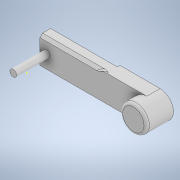
# Autodesk Inventor part: s.Strikrt
Saved by Autodesk Inventor 2020 (Build 240168000, 168)
## iProperties
Created: 2020-04-14
Part Number: s.Strikrt
Material: Generic
Document SubType Name: Modeling
Designer: Darugar
Density: 1 g/cm^3
Appearance: Default
Author: Darugar
Autodesk Inventor part; units mm, degrees
ref_plane "YZ Plane" through (0, 0, 0) normal (1, 0, 0) x (0, 1, 0)
ref_plane "XZ Plane" through (0, 0, 0) normal (0, 1, 0) x (-1, 0, 0)
ref_plane "XY Plane" through (0, 0, 0) normal (0, 0, 1) x (1, 0, 0)
sketch "Sketch1" plane through (0, 0, 0) normal (0, 0, 1) x (1, 0, 0)
  point P0 (0, 0)
sketch "Sketch2" plane through (0, 0, 0) normal (0, 0, 1) x (1, 0, 0)
  line L0 (0, 0) -> (50, 0)
  line L1 (50, 0) -> (50, 20)
  line L2 (50, 20) -> (0, 20)
  line L3 (0, 20) -> (0, 0)
  dimension "d0" = 50
  dimension "d1" = 20
  constraints: 8 end point, 2 parallel, 1 horizontal, 1 perpendicular
  measures "d0" distance of L2.end L1.end
  measures "d1" distance of L1.end L0.end
extrude "Extrusion1" add sketch "Sketch2" along normal blind 10
sketch "Sketch3" plane through (0, 0, 10) normal (0, 0, 1) x (1, 0, 0)
  line L0 (0, 20) -> (0, 0) projected
  line L1 (0, 10) -> (5, 10)
  circle A0 centre (5, 10) radius 2.5
  dimension "d4" = 5
  dimension "d5" = 5
  constraints: 2 end point, 1 centre point, 1 coincident, 1 horizontal, 1 midpoint
  measures "d4" distance of L1.start L1.end
  measures "d5" diameter of A0
extrude "Extrusion2" add sketch "Sketch3" along normal blind 25
sketch "Sketch4" plane through (0, 0, 10) normal (0, 0, 1) x (1, 0, 0)
  line L0 (50, 0) -> (50, 20) projected
  circle A0 centre (50, 10) radius 10
  point P0 (0, 0)
  dimension "d8" = 20
  constraints: 1 centre point, 1 midpoint
  measures "d8" diameter of A0
extrude "Extrusion3" add sketch "Sketch4" against normal blind 10 contours L0 A0 picked at (52.0783, 7.3939)
sketch "Sketch5" plane through (0, 0, 10) normal (0, 0, 1) x (1, 0, 0)
  line L0 (50, 20) -> (0, 20) projected
  line L1 (50, 20) -> (50, 10)
  line L2 (50, 20) -> (60, 20) construction
  circle A0 centre (50, 10) radius 10
  point P0 (0, 0)
  dimension "d11" = 10
  dimension "d12" = 90
  dimension "d13" = 20
  constraints: 4 end point, 1 centre point, 1 coincident, 1 horizontal, 1 perpendicular, 1 vertical
  measures "d11" distance of L0.start L1.end
  measures "d12" angle of L1 L2
  measures "d13" diameter of A0
extrude "Extrusion4" add sketch "Sketch5" along normal blind 10
chamfer "Chamfer1" distance 2 angle 45 5 edges at (40, 10, 20) (60, 10, 0) (25, 0, 0) (25, 20, 0) (25, 20, 10)
sketch "Sketch6" plane through (50, 10, 20) normal (0, 0, 1) x (1, 0, 0)
  point P0 (-50, -10)
sketch "Sketch7" plane through (50, 10, 20) normal (0, 0, 1) x (1, 0, 0)
  circle A0 centre (0, 0) radius 10
  point P0 (-50, -10)
  dimension "d19" = 20
  constraints: 1 centre point
  measures "d19" diameter of A0
extrude "Extrusion5" cut sketch "Sketch7" against normal blind 10
sketch "Sketch8" plane through (0, 0, 10) normal (0, 0, 1) x (1, 0, 0)
  arc A0 (50, 20) -> (44, 18) centre (50, 10) ccw projected
  line L0 (50, 20) -> (80, 20)
  line L1 (80, 20) -> (80, 0)
  line L2 (80, 0) -> (50, 0)
  line L3 (50, 0) -> (50, 20)
  point P0 (0, 0)
  dimension "d22" = 30
  constraints: 8 end point, 2 parallel, 1 horizontal, 1 perpendicular
  measures "d22" distance of L1.end L2.end
extrude "Extrusion6" add sketch "Sketch8" against normal blind 10
sketch "Sketch9" plane through (0, 0, 10) normal (0, 0, 1) x (1, 0, 0)
  line L0 (80, 20) -> (80, 0) projected
  circle A0 centre (80, 10) radius 10
  point P0 (0, 0)
  dimension "d25" = 20
  constraints: 1 centre point, 1 midpoint
  measures "d25" diameter of A0
extrude "Extrusion7" add sketch "Sketch9" against normal blind 10
sketch "Sketch10" plane through (0, 0, 10) normal (0, 0, 1) x (1, 0, 0)
  arc A0 (80, 0) -> (80, 20) centre (80, 10) ccw projected
  circle A1 centre (80, 10) radius 10
  point P0 (0, 0)
  point P1 (80, 20)
  point P2 (80, 0)
  dimension "d28" = 20
  constraints: 1 centre point, 1 coincident
  measures "d28" diameter of A1
extrude "Extrusion8" add sketch "Sketch10" along normal blind 10
fillet "Fillet1" radius 2 2 edges at (70, 10, 20) (90, 10, 20)
fillet "Fillet2" radius 2 1 edges at (46.8377, 19.4868, 8.5132)
body "Solid1"
